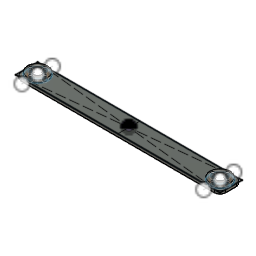
lab1-link_rr v3 (Autodesk Fusion 360 design; units mm, degrees)
Autodesk Fusion 360 part; units mm, degrees
sketch "Sketch1" plane through (0, 0, 0) normal (0, 0, 1) x (1, 0, 0)
  line L0 (112, 12) -> (-112, 12)
  line L1 (-112, 12) -> (-112, -12)
  line L2 (-112, -12) -> (112, -12)
  line L3 (112, -12) -> (112, 12)
  line L4 (112, 12) -> (-112, -12) construction
  line L5 (-112, 12) -> (112, -12) construction
  circle A0 centre (-100, 0) radius 11
  circle A1 centre (-100, 0) radius 8 construction
  circle A2 centre (-100, 0) radius 5
  line L6 (0, 12) -> (0, -12) construction
  circle A3 centre (100, 0) radius 11
  circle A4 centre (100, 0) radius 8 construction
  circle A5 centre (100, 0) radius 5
  line L7 (-100, 16) -> (-100, -17.1313) construction
  line L8 (100, 15) -> (100, -17.9102) construction
  circle A6 centre (-100, 8) radius 1.5
  circle A7 centre (-92, 0) radius 1.5
  circle A8 centre (-100, -8) radius 1.5
  circle A9 centre (-108, 0) radius 1.5
  circle A10 centre (100, 8) radius 1.5
  circle A11 centre (108, 0) radius 1.5
  circle A12 centre (92, 0) radius 1.5
  circle A13 centre (100, -8) radius 1.5
  dimension "d1" = 224
  dimension "d2" = 24
  dimension "d3" = 22
  dimension "d4" = 16
  dimension "d5" = 10
  dimension "d6" = 12
  dimension "d7" = 12
  dimension "d8" = 3
  dimension "d9" = 3
  dimension "d10" = 3
  dimension "d11" = 3
  dimension "d12" = 3
  dimension "d13" = 3
  dimension "d14" = 3
  dimension "d15" = 3
  constraint horizontal L0
  constraint perpendicular L0 L1
  constraint parallel L0 L2
  constraint parallel L1 L3
  constraint coincident L4 origin
  constraint coincident L5 origin
  constraint concentric A0 A1
  constraint concentric A1 A2
  constraint midpoint L0 L6.start
  constraint midpoint L2 L6.end
  constraint symmetric A0 L6 A3
  constraint symmetric A1 L6 A4
  constraint symmetric A2 L6 A5
  constraint vertical L7
  constraint perpendicular L0 L8
  constraint coincident A1 A6.centre
  constraint coincident L7 A6.centre
  constraint coincident A1 A7.centre
  constraint coincident L7 A8.centre
  constraint coincident A1 A8.centre
  constraint coincident A1 A9.centre
  constraint coincident A4 A10.centre
  constraint coincident L8 A10.centre
  constraint coincident A4 A11.centre
  constraint coincident A4 A12.centre
  constraint coincident A4 A13.centre
  constraint coincident L8 A13.centre
  measures "d1" distance of L0.start L0.end
  measures "d2" distance of L0.start L2.end
  measures "d3" diameter of A0
  measures "d4" diameter of A1
  measures "d5" diameter of A2
  measures "d6" distance of L1 L7
  measures "d7" distance of L3 L8
  measures "d8" diameter of A6
  measures "d9" diameter of A7
  measures "d10" diameter of A8
  measures "d11" diameter of A9
  measures "d12" diameter of A10
  measures "d13" diameter of A11
  measures "d14" diameter of A12
  measures "d15" diameter of A13
sketch "Sketch2" plane through (0, 0, 0) normal (0, 0, 1) x (1, 0, 0)
extrude "Extrude1" add sketch "Sketch1" along normal blind 3 contours A0 | A3 makes body 1 at (-106.962, -3.4918, 0) makes body 2 at (106.962, -3.4918, 0)
extrude "Extrude2" add sketch "Sketch1" against normal blind 3 separate body contours L0 L1 L2 L3 makes body 3
fillet "Fillet1" radius 6 2 edges at (-112, -12, -1.5) (112, -12, -1.5) on bodies 3
fillet "Fillet2" radius 6 2 edges at (112, 12, -1.5) (-112, 12, -1.5) on bodies 3
